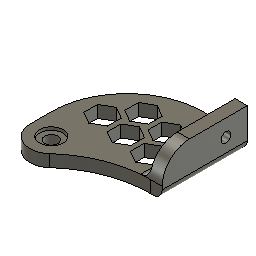
powersupply_side_support (Autodesk Fusion 360 design; units mm, degrees)
Autodesk Fusion 360 part; units mm, degrees
sketch "Sketch1" plane through (0, 0, 0) normal (0, 1, 0) x (1, 0, 0)
  line L0 (0, 0) -> (0, -46.4169) construction
  circle A0 centre (0, -32) radius 2.15
  line L1 (32.5, -28) -> (32.5, 0)
  line L2 (18, 0) -> (32.5, 0)
  circle A1 centre (0, -32) radius 3.85
  line L3 (-7, -32) -> (-7, -25)
  line L4 (32.5, -28) -> (28.5, -28)
  line L5 (28.5, -28) -> (28.5, -56.2606) construction
  arc A2 (28.5, -28) -> (4.7029, -37.1849) centre (28.5, -63.4206) ccw
  arc A3 (-7, -32) -> (4.7029, -37.1849) centre (0, -32) ccw
  arc A4 (18, 0) -> (-7, -25) centre (18, -25) ccw
  line L6 (18, -7.5) -> (14.1029, -9.75)
  line L7 (14.1029, -9.75) -> (14.1029, -14.25)
  line L8 (14.1029, -14.25) -> (18, -16.5)
  line L9 (18, -16.5) -> (21.8971, -14.25)
  line L10 (21.8971, -14.25) -> (21.8971, -9.75)
  line L11 (21.8971, -9.75) -> (18, -7.5)
  line L12 (11.8058, -14.7713) -> (7.9087, -17.0213)
  line L13 (7.9087, -17.0213) -> (7.9087, -21.5213)
  line L14 (7.9087, -21.5213) -> (11.8058, -23.7713)
  line L15 (11.8058, -23.7713) -> (15.7029, -21.5213)
  line L16 (15.7029, -21.5213) -> (15.7029, -17.0213)
  line L17 (15.7029, -17.0213) -> (11.8058, -14.7713)
  line L18 (21.2, -16.5) -> (17.3029, -18.75)
  line L19 (17.3029, -18.75) -> (17.3029, -23.25)
  line L20 (17.3029, -23.25) -> (21.2, -25.5)
  line L21 (21.2, -25.5) -> (25.0971, -23.25)
  line L22 (25.0971, -23.25) -> (25.0971, -18.75)
  line L23 (25.0971, -18.75) -> (21.2, -16.5)
  line L24 (4.7087, -8.0213) -> (4.7087, -12.5213)
  line L25 (4.7087, -12.5213) -> (8.6058, -14.7713)
  line L26 (8.6058, -14.7713) -> (12.5029, -12.5213)
  line L27 (12.5029, -12.5213) -> (12.5029, -8.0213)
  line L28 (12.5029, -8.0213) -> (8.6058, -5.7713)
  line L29 (8.6058, -5.7713) -> (4.7087, -8.0213)
  line L30 (-1.4856, -15.2926) -> (-1.4856, -19.7926)
  line L31 (-1.4856, -19.7926) -> (2.4115, -22.0426)
  line L32 (2.4115, -22.0426) -> (6.3087, -19.7926)
  line L33 (6.3087, -19.7926) -> (6.3087, -15.2926)
  line L34 (6.3087, -15.2926) -> (2.4115, -13.0426)
  line L35 (2.4115, -13.0426) -> (-1.4856, -15.2926)
  point P0 (18, -12)
  point P1 (11.8058, -19.2713)
  point P2 (21.2, -21)
  point P3 (8.6058, -10.2713)
  point P4 (2.4115, -17.5426)
  dimension "d1" = 4.3
  dimension "d2" = 32
  dimension "d3" = 32.5
  dimension "d4" = 7.7
  dimension "d5" = 14
  dimension "d6" = 28
  dimension "d17" = 4
  dimension "d28" = 50
  dimension "d29" = 4.5
  dimension "d30" = 14.5
  dimension "d31" = 12
  dimension "d32" = 4.5
  dimension "d33" = 1.6
  dimension "d34" = 1.6
  dimension "d35" = 4.5
  dimension "d36" = 1.6
  dimension "d37" = 1.6
  dimension "d38" = 4.5
  dimension "d39" = 1.6
  dimension "d40" = 1.6
  dimension "d41" = 4.5
  dimension "d42" = 1.6
  dimension "d43" = 1.6
  constraint coincident L0.start origin
  constraint vertical L0
  constraint coincident L0 A0.centre
  constraint vertical L1
  constraint perpendicular L1 L2
  constraint concentric A0 A1
  constraint concentric A0 A3
  constraint vertical L3
  constraint tangent L3 A3
  constraint perpendicular L1 L4
  constraint tangent L4 A2
  constraint tangent A2 A3
  constraint perpendicular L4 L5
  constraint coincident A2.centre L5
  constraint tangent L2 A4
  constraint tangent L3 A4
  constraint vertical L7
  constraint parallel L7 L16
  constraint parallel L16 L19
  constraint parallel L7 L27
  constraint parallel L7 L30
  measures "d1" diameter of A0
  measures "d2" distance of L0.start A0.centre
  measures "d3" distance of L0 L1
  measures "d4" diameter of A1
  measures "d5" diameter of A3
  measures "d6" distance of L1.end L1.start
  measures "d17" distance of L1.start L4.end
  measures "d28" diameter of A4
  measures "d29" distance of L6.start P0
  measures "d30" distance of L1 P0
  measures "d31" vertical distance of L0.start P0
  measures "d32" distance of L12.start P1
  measures "d33" distance of L8 L17
  measures "d34" distance of L7 L16
  measures "d35" distance of L18.start P2
  measures "d36" distance of L16 L19
  measures "d37" distance of L9 L18
  measures "d38" distance of L24.start P3
  measures "d39" distance of L12 L26
  measures "d40" distance of L7 L27
  measures "d41" distance of L30.start P4
  measures "d42" distance of L13 L33
  measures "d43" distance of L25 L34
extrude "Extrude1" add sketch "Sketch1" along normal blind 4 contours L1 L2 L3 L4 A2 A3 A4 | A1
sketch "Sketch2" plane through (32.5, 0, 0) normal (1, 0, 0) x (0, 0, -1)
  line L0 (-28, 0) -> (0, 0)
  line L1 (0, 0) -> (0, 4)
  line L2 (0, 4) -> (-28, 4)
  circle A0 centre (-7, 7.5) radius 1.6
  circle A1 centre (-7, 7.5) radius 3.5
  line L3 (0, 4) -> (0, 13)
  line L4 (0, 13) -> (-24.4425, 13)
  line L5 (-28, 4) -> (-28, 0)
  arc A2 (-19, 13) -> (-28, 4) centre (-19, 4) ccw
  point P0 (-17, 13)
  dimension "d9" = 3.2
  dimension "d10" = 7
  dimension "d11" = 7
  dimension "d12" = 17
  dimension "d13" = 9
  constraint concentric A0 A1
  constraint tangent L2 A1
  constraint coincident L1.end L2.start
  constraint perpendicular L2 L3
  constraint horizontal L4
  constraint coincident P0 L4
  constraint coincident L2 A2.centre
  constraint tangent L5 A2
  constraint tangent L4 A2
  constraint coincident L4 A2.start
  measures "d9" diameter of A0
  measures "d10" horizontal distance of L0.end A0.centre
  measures "d11" diameter of A1
  measures "d12" horizontal distance of L3.end P0
  measures "d13" distance of L1.end L3.end
extrude "Extrude2" add sketch "Sketch2" against normal blind 4 contours A1 | L2 L3 L4 A2
fillet "Fillet1" radius 3 1 edges at (28.5, 4, 14)
fillet "Fillet1" radius 3 1 edges at (32.5, 0, 14)
extrude "Extrude3" cut sketch "Sketch1" along normal up to surface (1 mm away) from surface at 3 contours A1
extrude "Extrude4" cut sketch "Sketch2" against normal blind 5 from surface at -3 contours A1
equation "d32 = d29"
equation "d34 = d33"
equation "d35 = d29"
equation "d36 = d33"
equation "d37 = d33"
equation "d38 = d29"
equation "d39 = d33"
equation "d40 = d33"
equation "d41 = d29"
equation "d42 = d33"
equation "d43 = d33"
